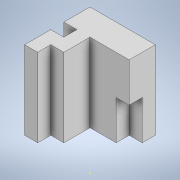
# Autodesk Inventor part: Martin-Probst-26673_obrazek_3
Saved by Autodesk Inventor 2021 (Build 250183000, 183)
## iProperties
Created: 2022-03-18
Part Number: Martin-Probst-26673_obrazek_3
Material: Všeobecné
Document SubType Name: Modeling
Designer: 26673
Density: 1 g/cm^3
Appearance: Výchozí
Author: 26673
Autodesk Inventor part; units mm, degrees
ref_plane "YZ Plane" through (0, 0, 0) normal (1, 0, 0) x (0, 1, 0)
ref_plane "XZ Plane" through (0, 0, 0) normal (0, 1, 0) x (-1, 0, 0)
ref_plane "XY Plane" through (0, 0, 0) normal (0, 0, 1) x (1, 0, 0)
sketch "Náčrt1" plane through (0, 0, 0) normal (1, 0, 0) x (0, 1, 0)
  line L0 (0, 0) -> (0, -50)
  line L1 (0, -50) -> (60, -50)
  line L2 (60, -50) -> (60, 0)
  line L3 (60, 0) -> (0, 0)
  dimension "d0" = 50
  dimension "d1" = 60
  constraints: 8 end point, 3 perpendicular, 1 vertical
  measures "d0" distance of L0.start L0.end
  measures "d1" distance of L0.end L1.end
extrude "Vysunutí1" add sketch "Náčrt1" along normal blind 50
sketch "Náčrt2" plane through (50, 0, 0) normal (1, 0, 0) x (0, 0, -1)
  line L0 (50, 0) -> (50, 60) projected
  line L1 (50, 60) -> (50, 30)
  line L2 (50, 30) -> (40, 30)
  line L3 (40, 30) -> (40, 0)
  line L4 (0, 0) -> (50, 0) projected
  line L5 (40, 0) -> (30, 0)
  line L6 (30, 0) -> (30, 30)
  line L7 (30, 30) -> (40, 30)
  dimension "d4" = 30
  dimension "d5" = 10
  dimension "d6" = 10
  constraints: 12 end point, 4 perpendicular, 3 point on line, 1 midpoint
  measures "d4" distance of L0.end L1.end
  measures "d5" distance of L1.end L2.end
  measures "d6" distance of L3.end L5.end
extrude "Vysunutí2" cut sketch "Náčrt2" against normal blind 10 contours L4 L6 L7 L3
sketch "Náčrt3" plane through (50, 0, 0) normal (1, 0, 0) x (0, 0, -1)
  point P0 (0, 0)
sketch "Náčrt4" plane through (50, 0, 0) normal (1, 0, 0) x (0, 0, -1)
  line L0 (0, 0) -> (30, 0) projected
  line L1 (0, 0) -> (30, 0)
  line L2 (30, 0) -> (30, 60)
  line L3 (50, 60) -> (0, 60) projected
  line L4 (0, 60) -> (0, 0) projected
  line L5 (30, 60) -> (0, 60)
  line L6 (0, 60) -> (0, 0)
  dimension "d9" = 30
  constraints: 8 end point, 2 perpendicular, 1 collinear, 1 horizontal, 1 point on line
  measures "d9" distance of L0.start L0.end
extrude "Vysunutí3" cut sketch "Náčrt4" against normal blind 30
sketch "Náčrt5" plane through (20, 0, 0) normal (1, 0, 0) x (0, 0, -1)
  line L0 (30, 0) -> (0, 0) projected
  line L1 (0, 0) -> (10, 0)
  line L2 (10, 0) -> (10, 60)
  line L3 (50, 60) -> (0, 60) projected
  line L4 (0, 60) -> (0, 0) projected
  line L5 (0, 60) -> (10, 60)
  line L6 (0, 60) -> (0, 0)
  dimension "d12" = 10
  constraints: 8 end point, 3 perpendicular, 2 point on line
  measures "d12" distance of L0.end L1.end
extrude "Vysunutí4" cut sketch "Náčrt5" against normal blind 10
sketch "Náčrt6" plane through (0, 0, 0) normal (-1, 0, 0) x (0, 0, 1)
  line L0 (-50, 60) -> (0, 60) projected
  line L1 (0, 60) -> (-20, 60)
  line L2 (-30, 60) -> (-30, 30) projected
  line L3 (-20, 60) -> (-30, 60)
  line L4 (-30, 0) -> (-30, 30) projected
  line L5 (-30, 60) -> (-30, 0)
  line L6 (-30, 0) -> (-20, 0)
  line L7 (-30, 0) -> (-10, 0) projected
  line L8 (-20, 0) -> (-20, 60)
  point P0 (0, 0)
  dimension "d15" = 20
  dimension "d16" = 10
  constraints: 10 end point, 1 collinear, 1 midpoint, 1 perpendicular, 1 point on line
  measures "d15" distance of L0.end L1.end
  measures "d16" distance of L4.start L6.end
extrude "Vysunutí5" cut sketch "Náčrt6" against normal blind 10
